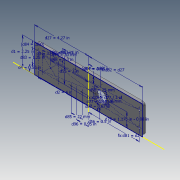
# Autodesk Inventor part: FLUGGER FLAT LOCK BRACKET
Saved by Autodesk Inventor 2020.3 (Build 243373000, 373)
## iProperties
RuleStatus: InUse
AfterDocSave0: file://Part Number Cleaner
Created: 2020-01-22
Material: Generic
Vendor: HHMI: JRC - ID&F
Document SubType Name: Modeling
Designer: arnoldj
Density: 1 g/cm^3
Appearance: Default
DESIGN DEPARTMENT: HHMI: JRC - ID&F
ALTERED ITEM PART NUMBER: N/A
ALTERED ITEM VENDOR: N/A
ALTERED ITEM DESCRIPTION: N/A
Author: arnoldj
Revision Number: 0
Autodesk Inventor part; units mm, degrees
ref_plane "YZ Plane" through (0, 0, 0) normal (1, 0, 0) x (0, 1, 0)
ref_plane "XZ Plane" through (0, 0, 0) normal (0, 1, 0) x (-1, 0, 0)
ref_plane "XY Plane" through (0, 0, 0) normal (0, 0, 1) x (1, 0, 0)
sketch "Sketch1" plane through (0, 0, 0) normal (0, 0, 1) x (1, 0, 0)
  line L0 (0, 68.58) -> (0, -11.43) projected
  line L1 (-151.8412, 0) -> (151.8412, 0) projected
  line L2 (108.458, 57.15) -> (-108.458, 57.15)
  line L3 (-108.458, 57.15) -> (-108.458, 0)
  line L4 (-108.458, 0) -> (108.458, 0)
  line L5 (108.458, 0) -> (108.458, 57.15)
  line L6 (-59.7, 12.7) -> (-92.7, 12.7) construction
  line L7 (-92.7, 12.7) -> (-92.7, 42.7) construction
  line L8 (-92.7, 42.7) -> (-59.7, 42.7) construction
  line L9 (-59.7, 42.7) -> (-59.7, 12.7) construction
  line L10 (-59.7, 12.7) -> (-92.7, 42.7) construction
  line L11 (-92.7, 12.7) -> (-59.7, 42.7) construction
  line L12 (11.884, 17.813) -> (36.884, 17.813) construction
  line L13 (36.884, 17.813) -> (36.884, 37.813) construction
  line L14 (36.884, 37.813) -> (11.884, 37.813) construction
  line L15 (11.884, 37.813) -> (11.884, 17.813) construction
  line L16 (11.884, 17.813) -> (36.884, 37.813) construction
  line L17 (36.884, 17.813) -> (11.884, 37.813) construction
  line L18 (101.6, 44.45) -> (-101.6, 44.45) construction
  line L19 (-101.6, 44.45) -> (-101.6, 12.7) construction
  line L20 (-101.6, 12.7) -> (101.6, 12.7) construction
  line L21 (101.6, 12.7) -> (101.6, 44.45) construction
  line L22 (101.6, 44.45) -> (-101.6, 12.7) construction
  line L23 (-101.6, 44.45) -> (101.6, 12.7) construction
  line L24 (-13.13, 17.018) -> (-35.13, 17.018) construction
  point P0 (0, 0)
  point P1 (101.6, 12.7)
  point P2 (-76.2, 27.7)
  point P3 (24.384, 27.813)
  point P4 (39.0271, 27.7128)
  point P5 (9.7409, 27.827)
  point P6 (-26.68, 49.53)
  point P7 (-52.08, 49.53)
  point P8 (0, 28.575)
  point P9 (-24.13, 17.018)
  dimension "d1" = 57.15
  dimension "d2" = 101.6
  dimension "d4" = 12.7
  dimension "d5" = 33
  dimension "d27" = 108.458
  dimension "d44" = 30
  dimension "d54" = 14.45
  dimension "d55" = 76.2
  dimension "d56" = 12.7
  dimension "d58" = 25
  dimension "d59" = 20
  dimension "d77" = 29.2862
  dimension "d78" = 14.6431
  dimension "d79" = 27.813
  dimension "d80" = 7.62
  dimension "d81" = 101.6
  dimension "d82" = 108.458
  dimension "d83" = 31.75
  dimension "d84" = 12.7
  dimension "d85" = 22
  dimension "d87" = 17.018
  dimension "d96" = 24.13
  dimension "d97" = 24.384
  dimension "d98" = 7.62
  dimension "d99" = 25.4
  constraints: 46 end point, 10 coincident, 8 midpoint, 8 parallel, 5 horizontal, 4 perpendicular, 2 horizontal alignment, 1 point on line
  measures "d1" distance of L2.end L3.end
  measures "d2" distance from line of L0 L19.end
  measures "d4" distance from line of L4 L19.end
  measures "d5" distance of L7.end L8.end
  measures "d27" distance between parallel lines of L3 L0
  measures "d44" distance of L8.end L6.start
  measures "d54" distance between parallel lines of L2 L8
  measures "d55" distance from line of L0 point (-76.2, 27.7)
  measures "d56" distance between parallel lines of L6 L1
  measures "d58" distance of L13.end L14.end
  measures "d59" distance of L12.end L13.end
  measures "d77" horizontal distance of point (9.741, 27.827) point (39.027, 27.713)
  measures "d78" horizontal distance of point (24.384, 27.813) point (39.027, 27.713)
  measures "d79" distance from line of point (24.384, 27.813) L1
  measures "d80" distance from line of L9 point (-52.08, 49.53)
  measures "d81" distance from line of point (101.6, 12.7) L0
  measures "d82" distance between parallel lines of L0 L5
  measures "d83" distance of L18.end L19.end
  measures "d84" distance between parallel lines of L18 L2
  measures "d85" distance of L24.start L24.end
  measures "d87" distance from line of L24.start L1
  measures "d96" distance from line of point (-24.13, 17.018) L0
  measures "d97" distance from line of L0 point (24.384, 27.813)
  measures "d98" distance from line of point (-52.08, 49.53) L2
  measures "d99" distance of point (-26.68, 49.53) point (-52.08, 49.53)
extrude "Extrusion1" add sketch "Sketch1" against normal blind 5.842
hole "Hole1" at (-101.6, 12.7, 0) at (101.6, 12.7, 0) at (-101.6, 44.45, 0) at (101.6, 44.45, 0) direction (0, 0, -1) diameter 5.461 end through all
sketch "Sketch3" plane through (0, 0, 0) normal (0, 0, 1) x (1, 0, 0)
  point P0 (0, 0)
hole "Hole4 Tap M3" at (-92.7, 42.7, 0) at (-59.7, 42.7, 0) at (-59.7, 12.7, 0) at (-92.7, 12.7, 0) at (-26.68, 49.53, 0) at (-52.08, 49.53, 0) direction (0, 0, -1) diameter 2.3622 end through all
fillet "Fillet2" radius 4.7498 4 edges at (-108.458, 57.15, -2.921) (108.458, 57.15, -2.921) (108.458, 0, -2.921) (-108.458, 0, -2.921)
hole "Hole5" at (36.884, 37.813, 0) at (36.884, 17.813, 0) at (11.884, 17.813, 0) at (11.884, 37.813, 0) at (39.0271, 27.7128, 0) at (9.7409, 27.827, 0) direction (0, 0, -1) diameter 2.3622 end through all
hole "Hole6" at (24.384, 27.813, 0) direction (0, 0, -1) diameter 22.86 end through all
hole "Hole7 Tap M4" at (-35.13, 17.018, 0) at (-13.13, 17.018, 0) direction (0, 0, -1) diameter 3.242 end through all thread size "M4x0.7" class "6H" standard "ANSI Metric M Profile"
mirror "Mirror1" about plane through (0, 0, 0) normal (1, 0, 0) of "Hole4 Tap M3"
equation "\"d78\" = 0.5 * d77"
equation "\"d81\" = d2"
equation "\"d82\" = d27"
body "Solid1"
